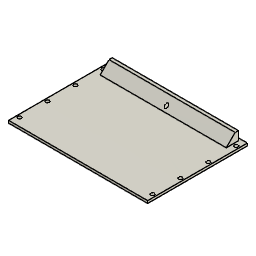
Rear Panel - Blank (Autodesk Fusion 360 design; units mm, degrees)
Autodesk Fusion 360 part; units mm, degrees
sketch "Sketch1" plane through (0, 0, 0) normal (0, 0, 1) x (1, 0, 0)
  line L0 (-86.3, -61.9) -> (86.3, -61.9)
  line L1 (86.3, -61.9) -> (86.3, 61.9)
  line L2 (86.3, 61.9) -> (-86.3, 61.9)
  line L3 (-86.3, 61.9) -> (-86.3, -61.9)
  point P0 (0, -61.9)
  point P1 (-86.3, 0)
  dimension "d1" = 172.6
  dimension "d2" = 123.8
  constraint horizontal L0
  constraint vertical L1
  constraint horizontal L2
  constraint vertical L3
  constraint midpoint L0 P0
  constraint midpoint L3 P1
  measures "d1" distance of L0.start L0.end
  measures "d2" distance of L0.start L2.end
extrude "Extrude1" add sketch "Sketch1" along normal blind 3
sketch "Sketch2" plane through (0, 0, 0) normal (0, 0, -1) x (1, 0, 0)
  line L0 (-86.3, 61.9) -> (-86.3, -61.9)
  line L1 (-86.3, -61.9) -> (86.3, -61.9)
  line L2 (86.3, -61.9) -> (86.3, 61.9)
  line L3 (86.3, 61.9) -> (-86.3, 61.9)
  line L4 (-82.5, 61.9) -> (-82.5, 55.1688)
  line L5 (-82.5, 55.1688) -> (-82.5, -61.9) construction
  line L6 (0, 61.9) -> (0, -61.9) construction
  line L7 (82.5, 61.9) -> (82.5, -61.9) construction
  line L8 (-86.3, 0) -> (-82.7712, 0)
  line L9 (-82.7712, 0) -> (86.3, 0) construction
  circle A0 centre (-82.5, 51.9) radius 2.25
  circle A1 centre (-82.5, 17.3) radius 2.25
  circle A2 centre (-82.5, -17.3) radius 2.25
  circle A3 centre (-82.5, -51.9) radius 2.25
  circle A4 centre (82.5, 51.9) radius 2.25
  circle A5 centre (82.5, 17.3) radius 2.25
  circle A6 centre (82.5, -17.3) radius 2.25
  circle A7 centre (82.5, -51.9) radius 2.25
  dimension "d5" = 3.8
  dimension "d6" = 3.8
  dimension "d7" = 4.5
  dimension "d8" = 4.5
  dimension "d9" = 4.5
  dimension "d10" = 4.5
  dimension "d11" = 4.5
  dimension "d12" = 4.5
  dimension "d13" = 4.5
  dimension "d14" = 4.5
  dimension "d15" = 10
  dimension "d16" = 10
  dimension "d17" = 34.6
  dimension "d18" = 34.6
  dimension "d19" = 34.6
  constraint coincident L3 L4.start
  constraint perpendicular L3 L4
  constraint coincident L1 L5.end
  constraint perpendicular L1 L5
  constraint midpoint L3 L6.start
  constraint midpoint L1 L6.end
  constraint coincident L3 L7.start
  constraint coincident L1 L7.end
  constraint perpendicular L1 L7
  constraint midpoint L0 L8.start
  constraint perpendicular L0 L8
  constraint midpoint L2 L9.end
  constraint perpendicular L2 L9
  constraint coincident L5 A0.centre
  constraint coincident L5 A1.centre
  constraint coincident L5 A2.centre
  constraint coincident L5 A3.centre
  constraint coincident L7 A4.centre
  constraint coincident L7 A5.centre
  constraint coincident L7 A6.centre
  constraint coincident L7 A7.centre
  constraint horizontal A0.centre A4.centre
  constraint horizontal A1.centre A5.centre
  constraint horizontal A2.centre A6.centre
  constraint horizontal A3.centre A7.centre
  measures "d5" distance of L0 L5
  measures "d6" distance of L2 L7
  measures "d7" diameter of A0
  measures "d8" diameter of A1
  measures "d9" diameter of A2
  measures "d10" diameter of A3
  measures "d11" diameter of A4
  measures "d12" diameter of A5
  measures "d13" diameter of A6
  measures "d14" diameter of A7
  measures "d15" distance of L3 A0.centre
  measures "d16" distance of L1 A3.centre
  measures "d17" distance of A0.centre A1.centre
  measures "d18" distance of A1.centre A2.centre
  measures "d19" distance of A2.centre A3.centre
extrude "Extrude2" cut sketch "Sketch2" against normal through all contours A0 | A1 | A2 | A3 | A4 | A5 | A6 | A7
sketch "Sketch4" plane through (0, 0, 3) normal (0, 0, 1) x (-1, 0, 0)
  circle A0 centre (-82.5, 17.3) radius 2.25
  circle A1 centre (82.5, 17.3) radius 2.25
  circle A2 centre (82.5, -17.3) radius 2.25
  circle A3 centre (-82.5, -17.3) radius 2.25
  circle A4 centre (-82.5, 51.9) radius 2.25
  circle A5 centre (82.5, 51.9) radius 2.25
  circle A6 centre (82.5, -51.9) radius 2.25
  circle A7 centre (-82.5, -51.9) radius 2.25
  line L0 (86.3, -61.9) -> (86.3, 61.9)
  line L1 (86.3, 61.9) -> (-86.3, 61.9)
  line L2 (-86.3, 61.9) -> (-86.3, -61.9)
  line L3 (-86.3, -61.9) -> (86.3, -61.9)
  line L4 (78.25, -58.7) -> (-78.25, -58.7)
  line L5 (-78.25, -58.7) -> (-78.25, -54.7)
  line L6 (-78.25, -54.7) -> (78.25, -54.7)
  line L7 (78.25, -54.7) -> (78.25, -58.7)
  dimension "d21" = 8.05
  dimension "d22" = 8.05
  dimension "d23" = 3.2
  dimension "d24" = 4
  constraint horizontal L4
  constraint vertical L5
  constraint horizontal L6
  constraint vertical L7
  measures "d21" distance of L0 L7
  measures "d22" distance of L2 L5
  measures "d23" distance of L3 L4
  measures "d24" distance of L4 L6
extrude "Extrude3" add sketch "Sketch4" along normal blind 11 contours L4 L5 L6 L7
chamfer "Chamfer1" distance 11 angle 45 1 edges at (0, 54.7, 3)
sketch "Sketch5" plane through (0, 58.7, 0) normal (0, 1, 0) x (-1, 0, 0)
  line L0 (-78.25, 3) -> (78.25, 3)
  line L1 (78.25, 3) -> (78.25, 14)
  line L2 (78.25, 14) -> (-78.25, 14)
  line L3 (-78.25, 14) -> (-78.25, 3)
  line L4 (-78.25, 7) -> (-74.8541, 7)
  line L5 (-74.8541, 7) -> (78.25, 7) construction
  circle A0 centre (0, 7) radius 1.95
  dimension "d28" = 4
  dimension "d29" = 3.9
  dimension "d30" = 78.25
  constraint coincident L3 L4.start
  constraint perpendicular L3 L4
  constraint coincident L1 L5.end
  constraint perpendicular L1 L5
  constraint coincident L5 A0.centre
  measures "d28" distance of L0 L5
  measures "d29" diameter of A0
  measures "d30" distance of L3 A0.centre
extrude "Extrude4" cut sketch "Sketch5" against normal blind 14 contours A0
equation "d6 = d5"
equation "d8 = d7"
equation "d9 = d7"
equation "d10 = d9"
equation "d11 = d7"
equation "d12 = d7"
equation "d13 = d7"
equation "d14 = d7"
equation "d18 = d17"
equation "d22 = d21"
